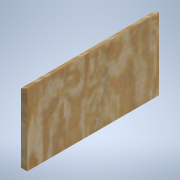
# Autodesk Inventor part: Back
Saved by Autodesk Inventor 2021.1 (Build 251245000, 245)
## iProperties
Created: 2020-08-02
Part Number: Back
Material: Generic
Document SubType Name: Modeling
Designer: adick
Density: 1 g/cm^3
Appearance: Default
Author: adick
Autodesk Inventor part; units mm, degrees
ref_plane "YZ Plane" through (0, 0, 0) normal (1, 0, 0) x (0, 1, 0)
ref_plane "XZ Plane" through (0, 0, 0) normal (0, 1, 0) x (-1, 0, 0)
ref_plane "XY Plane" through (0, 0, 0) normal (0, 0, 1) x (1, 0, 0)
sketch "Sketch1" plane through (0, 0, 0) normal (0, 0, 1) x (1, 0, 0)
  line L0 (135, 77) -> (135, -77) projected
  line L1 (135, -70.65) -> (-135, -70.65) projected
  line L2 (-35.423, -7) -> (135, 77) projected
  line L3 (-135, -7) -> (-35.423, -7) projected
  line L4 (135, -70.65) -> (129.3043, -70.65)
  line L5 (135, 73.4092) -> (135, -70.65)
  line L6 (135, -70.65) -> (129.3043, -70.65)
  line L7 (135, -7) -> (135, -70.65)
  line L8 (135, 77) -> (135, 73.4661)
  line L9 (135, 77) -> (129.3043, 74.1926)
  line L10 (135, -70.65) -> (122.3, -70.65)
  line L11 (122.3, -70.65) -> (122.3, 70.7403)
  line L12 (135, 70.7403) -> (135, -70.65)
  line L13 (129.3043, 74.1926) -> (122.3, 70.7403)
  point P0 (0, 0)
  constraints: 20 end point, 3 collinear, 3 horizontal, 3 point on line, 1 parallel, 1 perpendicular
extrude "Extrusion1" add sketch "Sketch1" along normal blind 270
body "Solid1"
